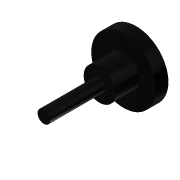
# Autodesk Inventor part: Knob
Saved by Autodesk Inventor 2014 (Build 180170000, 170)
## iProperties
Created: 2014-08-10
Part Number: Knob
Material: Generic
Document SubType Name: Modeling
Designer: Peele
Density: 1 g/cm^3
Appearance: Glossy - Black
Author: Peele
Autodesk Inventor part; units mm, degrees
ref_plane "YZ Plane" through (0, 0, 0) normal (1, 0, 0) x (0, 1, 0)
ref_plane "XZ Plane" through (0, 0, 0) normal (0, 1, 0) x (-1, 0, 0)
ref_plane "XY Plane" through (0, 0, 0) normal (0, 0, 1) x (1, 0, 0)
sketch "Sketch1" plane through (0, 0, 0) normal (0, 0, 1) x (1, 0, 0)
  line L0 (0, 0) -> (0, 73)
  line L1 (0, 73) -> (25.5, 73)
  line L2 (25.5, 73) -> (25.5, 63)
  line L3 (25.5, 63) -> (12.5, 63)
  line L4 (12.5, 63) -> (12.5, 44)
  line L5 (12.5, 44) -> (5, 44)
  line L6 (5, 44) -> (5, 0)
  line L7 (5, 0) -> (0, 0)
  dimension "d0" = 25.5
  dimension "d1" = 10
  dimension "d2" = 19
  dimension "d3" = 12.5
  dimension "d4" = 44
  dimension "d5" = 5
  constraints: 16 end point, 6 parallel, 1 perpendicular, 1 vertical
  measures "d0" distance between parallel lines of L0 L2
  measures "d1" distance of L1.end L2.end
  measures "d2" distance of L3.end L4.end
  measures "d3" distance between parallel lines of L0 L4
  measures "d4" distance of L5.end L6.end
  measures "d5" distance of L6.end L0.start
revolve "Revolution1" add sketch "Sketch1" angle 360 about axis through (0, 0, 0) along (0, 1, 0)
body "Solid1"
